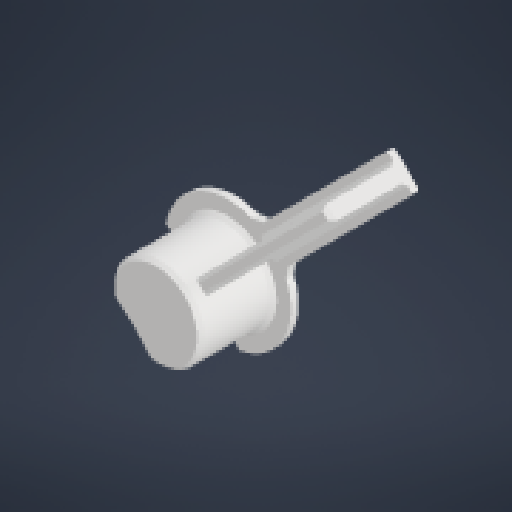
# Autodesk Inventor part: HourGuard_36_wavyV2
Saved by Autodesk Inventor 2023.1 (Build 271208000, 208)
## iProperties
Created: 2023-08-28
Part Number: HourGuard_36_wavyV2
Material: Generic
Document SubType Name: Modeling
Designer: washichi
Density: 1 g/cm^3
Appearance: Default
Author: washichi
## iProperties of the stored document HourGuard_36_wavyV2_3DPrint.ipt
Created: 2023-08-28
Part Number: HourGuard_36_wavyV2_3DPrint
Material: Generic
Document SubType Name: Modeling
Designer: washichi
Density: 1 g/cm^3
Appearance: Default
Author: washichi
Autodesk Inventor part; units mm, degrees
ref_plane "YZ Plane" through (0, 0, 0) normal (1, 0, 0) x (0, 1, 0)
ref_plane "XZ Plane" through (0, 0, 0) normal (0, 1, 0) x (-1, 0, 0)
ref_plane "XY Plane" through (0, 0, 0) normal (0, 0, 1) x (1, 0, 0)
sketch "Sketch3" plane through (0, 0, 0) normal (0, 0, 1) x (1, 0, 0)
  line L0 (0, 0) -> (103.9447, 103.9447)
  line L1 (0, 0) -> (147, 0) construction
  arc A0 (67.2085, 42.6098) -> (42.6098, 67.2085) centre (0, 0) ccw
  circle A1 centre (56.2698, 56.2698) radius 17.5
  circle A2 centre (0, 0) radius 71
  line L2 (67.2085, 42.6098) -> (63.0672, 32.6118)
  line L3 (67.2085, 42.6098) -> (78.0302, 42.6098) construction
  line L4 (42.6098, 67.2085) -> (32.6118, 63.0672)
  line L5 (42.6098, 67.2085) -> (53.4315, 67.2085) construction
  line L6 (106.7731, 99.7021) -> (12.0711, 5)
  line L7 (12.0711, 5) -> (147, 5)
  line L8 (99.7021, 106.7731) -> (-12.0711, -5)
  line L9 (-12.0711, -5) -> (147, -5)
  line L10 (103.9447, 103.9447) -> (101.1163, 106.7731)
  line L11 (103.9447, 103.9447) -> (106.7731, 101.1163)
  arc A3 (101.1163, 106.7731) -> (99.7021, 106.7731) centre (100.4092, 106.066) ccw
  arc A4 (106.7731, 99.7021) -> (106.7731, 101.1163) centre (106.066, 100.4092) ccw
  point P0 (71.6638, 64.5928)
  point P1 (64.5928, 71.6638)
  point P2 (68.6441, 68.6441)
  point P3 (70.8237, -5)
  point P4 (40.8757, 47.9468)
  point P5 (39.0352, 59.3064)
  point P6 (46.5444, 53.6155)
  point P7 (70.8237, 5)
  point P8 (47.9468, 40.8757)
  point P9 (53.6155, 46.5444)
  point P10 (59.3064, 39.0352)
  point P11 (43.8954, 43.8954)
  point P12 (50.2046, 50.2046)
  dimension "d26" = 147
  dimension "d27" = 45
  dimension "d28" = 159.1549
  dimension "d29" = 35
  dimension "d30" = 142
  dimension "d31" = 112.5
  dimension "d32" = 157.5
  dimension "d33" = 5
  dimension "d34" = 5
  dimension "d35" = 1
  constraints: 24 end point, 11 point on circle, 5 centre point, 4 tangent, 3 equal length, 3 horizontal, 2 coincident, 1 equal radius, 1 point on line, 2 other
  measures "d26" distance of L0.start L0.end
  measures "d27" angle of L1 L0
  measures "d28" diameter of A0
  measures "d29" diameter of A1
  measures "d30" diameter of A2
  measures "d31" angle of L2 L3
  measures "d32" angle of L4 L5
  measures "d33" distance between parallel lines of L0 L6
  measures "d34" distance between parallel lines of L0 L8
  measures "d35" radius of A3
extrude "Extrusion2" add sketch "Sketch3" along normal blind 2 contours A2 L8 A0 L0 | L0 A0 L6 A2 | A0 L8 A1 L0 | L0 A1 L6 A0 | L6 A0 A1 A2 | A2 A1 A0 L8 | A1 L8 A3 L10 L0 | L0 L11 A4 L6 A1 | L6 A1 A0 | A0 A1 L8
sketch "Sketch4" plane through (0, 0, 2) normal (0, 0, 1) x (1, 0, 0)
  arc A0 (64.5928, 71.6638) -> (39.0352, 59.3064) centre (56.2698, 56.2698) ccw projected
  arc A1 (59.3064, 39.0352) -> (71.6638, 64.5928) centre (56.2698, 56.2698) ccw projected
  circle A2 centre (56.2698, 56.2698) radius 12.5
  line L0 (56.2698, 56.2698) -> (103.9447, 103.9447)
  line L1 (54.8556, 57.684) -> (102.5305, 105.3589)
  line L2 (57.684, 54.8556) -> (105.3589, 102.5305)
  line L3 (71.6638, 64.5928) -> (64.5928, 71.6638)
  circle A3 centre (56.2698, 56.2698) radius 7.5
  arc A4 (59.3064, 39.0352) -> (39.0352, 59.3064) centre (0, 0) ccw projected
  arc A5 (65.732, 33.9898) -> (33.9898, 65.732) centre (0, 0) ccw
  line L4 (103.9447, 103.9447) -> (105.3589, 102.5305)
  line L5 (106.7731, 101.1163) -> (101.1163, 106.7731) projected
  line L6 (102.5305, 105.3589) -> (103.9447, 103.9447)
  circle A6 centre (0, 0) radius 93.5775
  circle A7 centre (56.2698, 56.2698) radius 17.5
  point P0 (42.6098, 67.2085)
  point P1 (67.2085, 42.6098)
  point P2 (32.6118, 63.0672)
  point P3 (63.0672, 32.6118)
  point P4 (69.5425, 66.7141)
  point P5 (66.7141, 69.5425)
  point P6 (43.7753, 55.8993)
  point P7 (55.8993, 43.7753)
  point P8 (51.9915, 48.3517)
  point P9 (48.3517, 51.9915)
  point P10 (55.6314, 48.797)
  point P11 (48.797, 55.6314)
  dimension "d38" = 25
  dimension "d39" = 2
  dimension "d40" = 2
  dimension "d41" = 5
  dimension "d56" = 3
  dimension "d66" = 187.1549
  dimension "d67" = 35
  constraints: 12 end point, 5 centre point, 3 coincident, 2 collinear, 2 parallel, 2 point on circle
  measures "d38" diameter of A2
  measures "d39" distance between parallel lines of L0 L1
  measures "d40" distance between parallel lines of L0 L2
  measures "d41" radial gap between concentric circles of A2 A3
  measures "d56" radial gap between concentric circles of A4 A5
  measures "d66" diameter of A6
  measures "d67" diameter of A7
extrude "Extrusion3" add sketch "Sketch4" along normal blind 20 contours L1 A7 L0 L3 | L1 L5 L0 A7 | L0 A7 L2 L3 | L0 L4 L2 A7 | A5 A3 A2 A4 | A2 L1 A3 A5 | A2 L0 A3 L1 | A5 A3 | A3 A5 | A2 L2 A3 L0 | A3 L2 A2 A5
chamfer "Chamfer6" distance 1 angle 45 9 edges at (68.1283, 68.1283, 2) (65.1086, 65.1086, 22) (84.6223, 87.4507, 22) (87.4507, 84.6223, 22) (68.1283, 68.1283, 22) (103.9447, 103.9447, 22) (84.6223, 87.4507, 2) (87.4507, 84.6223, 2) (65.1086, 65.1086, 2)
chamfer "Chamfer7" distance 2 angle 45 2 edges at (64.5928, 71.6638, 1) (71.6638, 64.5928, 1)
body "Solid2"
